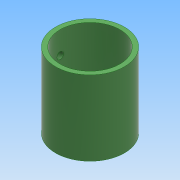
# Autodesk Inventor part: Top_Separator Pipe
Saved by Autodesk Inventor 2018.1 (Build 221171000, 171)
## iProperties
Created: 2019-02-25
Part Number: Top_Separator Pipe
Material: PVC-Piping
Document SubType Name: Modeling
Designer: James
Density: 1.4 g/cm^3
Appearance: Smooth - Dark Forest Green
Author: James
Autodesk Inventor part; units mm, degrees
ref_plane "YZ Plane" through (0, 0, 0) normal (1, 0, 0) x (0, 1, 0)
ref_plane "XZ Plane" through (0, 0, 0) normal (0, 1, 0) x (-1, 0, 0)
ref_plane "XY Plane" through (0, 0, 0) normal (0, 0, 1) x (1, 0, 0)
sketch "Sketch1" plane through (0, 0, 0) normal (0, 0, 1) x (1, 0, 0)
  circle A0 centre (0, 0) radius 20
  circle A1 centre (0, 0) radius 23
  dimension "d0" = 40
  dimension "d1" = 46
  constraints: 2 centre point, 2 coincident
  measures "d0" diameter of A0
  measures "d1" diameter of A1
extrude "Extrusion1" add sketch "Sketch1" along normal mid plane 50
sketch "Sketch2" plane through (0, 0, 0) normal (1, 0, 0) x (0, 1, 0)
  line L0 (0, 105) -> (0, -105) projected
  line L1 (-105, 0) -> (105, 0) projected
  line L2 (23, 25) -> (-23, 25) projected
  line L3 (-23, -25) -> (23, -25) projected
  point P0 (0, 0)
  point P1 (0, 10)
  point P2 (0, -10)
  point P3 (0, -25)
  dimension "d21" = 20
  dimension "d22" = 15
  constraints: 2 vertical alignment, 1 midpoint
  measures "d21" distance of point (0, -10) point (0, 10)
  measures "d22" distance from line of L2 point (0, 10)
hole "Hole1" at (0, 0, 10) at (0, 0, -10) direction (-1, 0, 0) diameter 4.5 end through all clearance for "Flat Head Machine Screw" size "M4" standard "Ansi Metric M Profile"
sketch "Sketch3" plane through (0, 0, 0) normal (1, 0, 0) x (0, 1, 0)
  line L0 (23, -25) -> (7, -25)
  line L1 (7, -25) -> (7, 25)
  line L2 (7, 25) -> (23, 25)
  line L3 (23, 25) -> (23, -25)
  line L4 (23, 25) -> (-23, 25) projected
  line L5 (-23, -25) -> (23, -25) projected
  line L6 (0, 195.3) -> (0, -195.3) projected
  point P0 (0, 0)
  dimension "d13" = 0
  dimension "d14" = 0
  dimension "d15" = 7
  constraints: 8 end point, 2 parallel, 1 coincident, 1 horizontal, 1 perpendicular
  measures "d13" distance between parallel lines of L4 L2
  measures "d14" distance between parallel lines of L5 L0
  measures "d15" distance between parallel lines of L6 L1
extrude "Extrusion2" [suppressed]
body "Solid1"
